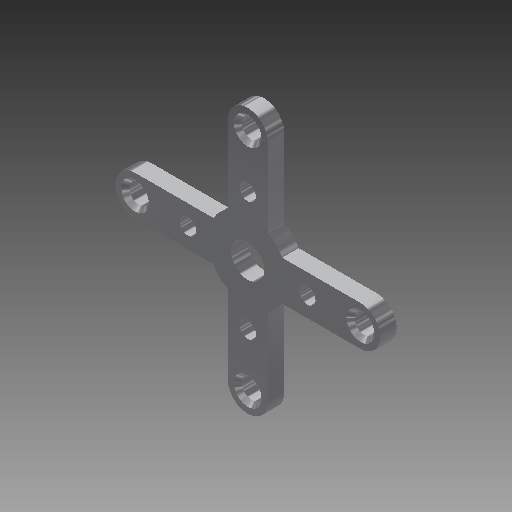
# Autodesk Inventor part: HK 2830 mounting plate
Saved by Autodesk Inventor 2019 (Build 230136000, 136)
## iProperties
Created: 2014-01-18
Part Number: HK 2830 mounting plate
Document SubType Name: Modeling
Designer: Phil
Density: 1 g/cm^3
Material: Generic
Appearance: Aluminum - Polished
Author: Phil
Autodesk Inventor part; units mm, degrees
ref_plane "YZ Plane" through (0, 0, 0) normal (1, 0, 0) x (0, 1, 0)
ref_plane "XZ Plane" through (0, 0, 0) normal (0, 1, 0) x (-1, 0, 0)
ref_plane "XY Plane" through (0, 0, 0) normal (0, 0, 1) x (1, 0, 0)
sketch "Sketch2" plane through (0, 0, 0) normal (0, 0, 1) x (1, 0, 0)
  circle A0 centre (0, 0) radius 2.5
  circle A1 centre (0, 0) radius 6
  dimension "d12" = 5
  dimension "d13" = 12
  constraints: 2 centre point, 2 coincident
  measures "d12" diameter of A0
  measures "d13" diameter of A1
extrude "Extrusion1" add sketch "Sketch2" along normal blind 2.5
sketch "Sketch3" plane through (0, 0, 2.5) normal (0, 0, 1) x (1, 0, 0)
  circle A0 centre (0, 0) radius 2.5 projected
  circle A1 centre (0, 0) radius 6 projected
  line L0 (0, 0) -> (0, -18.3723) construction
  circle A2 centre (0, -17) radius 1.5
  circle A3 centre (0, -9) radius 1.25
  line L1 (3, -5.1962) -> (3, -17)
  line L2 (-3, -17) -> (-3, -5.1962)
  line L3 (5.4814, -17) -> (-5.6867, -17) construction
  arc A4 (-3, -17) -> (3, -17) centre (0, -17) ccw
  dimension "d16" = 3
  dimension "d17" = 2.5
  dimension "d18" = 9
  dimension "d19" = 17
  dimension "d20" = 3
  dimension "d21" = 3
  constraints: 8 end point, 4 point on circle, 4 point on line, 3 centre point, 2 parallel, 2 tangent, 1 perpendicular, 1 vertical
  measures "d16" diameter of A2
  measures "d17" diameter of A3
  measures "d18" distance of A3.centre A0.centre
  measures "d19" distance of A0.centre A2.centre
  measures "d20" distance between parallel lines of L0 L1
  measures "d21" distance between parallel lines of L2 L0
extrude "Extrusion2" add sketch "Sketch3" against normal blind 2.5 contours A1 L1 A4 L2
pattern_circular "Circular Pattern1" count 4 over 360 about axis through (0, 0, 0) along (0, 0, 1) of "Extrusion2"
chamfer "Chamfer1" distance 0.6 angle 45 4 edges at (-1.5, -17, 2.5) (17, -1.5, 2.5) (-17, 1.5, 2.5) (1.5, 17, 2.5)
equation "\"d21\" = d20"
body "Solid1"
